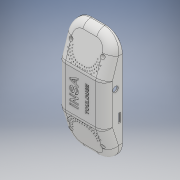
# Autodesk Inventor part: Partie basse
Saved by Autodesk Inventor 2019 (Build 230136000, 136)
## iProperties
Created: 2018-06-04
Part Number: Partie basse
Material: Plastique ABS
Document SubType Name: Modeling
Designer: dimercur
Mass: 82.847 g
Surface Area: 638.157 cm^2
Volume: 78.1576 cm^3
Density: 1.06 g/cm^3
Appearance: Lisse - Blanc
Author: dimercur
Autodesk Inventor part; units mm, degrees
ref_plane "YZ Plane" through (0, 0, 0) normal (1, 0, 0) x (0, 1, 0)
ref_plane "XZ Plane" through (0, 0, 0) normal (0, 1, 0) x (-1, 0, 0)
ref_plane "XY Plane" through (0, 0, 0) normal (0, 0, 1) x (1, 0, 0)
sketch "Esquisse1" plane through (0, 0, 0) normal (0, 1, 0) x (-1, 0, 0)
  line L0 (42.5, 100) -> (-42.5, 100)
  line L1 (-42.5, 100) -> (-42.5, -100)
  line L2 (-42.5, -100) -> (42.5, -100)
  line L3 (42.5, -100) -> (42.5, 100)
  point P0 (0, 0)
  dimension "d0" = 200
  dimension "d1" = 85
  dimension "d2" = 42.5
  dimension "d3" = 100
  constraints: 8 end point, 2 parallel, 1 horizontal, 1 perpendicular
  measures "d0" distance of L2.end L0.start
  measures "d1" distance of L0.start L0.end
  measures "d2" horizontal distance of point (0, 0) L0.start
  measures "d3" vertical distance of point (0, 0) L0.start
extrude "Extrusion1" add sketch "Esquisse1" along normal blind 34
sketch "Esquisse14" plane through (0, 34, 0) normal (0, 1, 0) x (1, 0, 0)
  circle A0 centre (-27.5, -70) radius 3.5
  circle A1 centre (29.5, -70) radius 3.5
  circle A2 centre (29.5, 70) radius 3.5
  circle A3 centre (-27.5, 70) radius 3.5
  line L0 (-42.5, 100) -> (-42.5, -100) projected
  line L1 (42.5, -100) -> (42.5, 100) projected
  line L2 (-42.5, -100) -> (42.5, -100) projected
  line L3 (42.5, 100) -> (-42.5, 100) projected
  point P0 (0, 0)
  dimension "d110" = 7
  dimension "d111" = 7
  dimension "d112" = 7
  dimension "d113" = 7
  dimension "d114" = 15
  dimension "d115" = 15
  dimension "d116" = 13
  dimension "d117" = 13
  dimension "d118" = 30
  dimension "d119" = 30
  dimension "d120" = 30
  dimension "d121" = 30
  constraints: 4 centre point
  measures "d110" diameter of A0
  measures "d111" diameter of A1
  measures "d112" diameter of A2
  measures "d113" diameter of A3
  measures "d114" distance from line of L0 A0.centre
  measures "d115" distance from line of L0 A3.centre
  measures "d116" distance from line of L1 A1.centre
  measures "d117" distance from line of L1 A2.centre
  measures "d118" distance from line of L2 A0.centre
  measures "d119" distance from line of L2 A1.centre
  measures "d120" distance from line of L3 A3.centre
  measures "d121" distance from line of L3 A2.centre
extrude "Extrusion11" cut sketch "Esquisse14" against normal through all contours A0 | A1 | A2 | A3
chamfer "Chanfrein1" distance 20 angle 72 1 edges at (0, 0, 100) measured on face at (0, 0.5, 100)
chamfer "Chanfrein2" distance 20 angle 72 1 edges at (0, 0, -100) measured on face at (0, 0.5, -100)
fillet "Congé3" radius 30 4 edges at (-42.5, 27, 100) (42.5, 27, 100) (-42.5, 27, -100) (42.5, 27, -100)
fillet "Congé4" radius 15 14 edges at (0, 0, 38.4463) (-33.7132, 17.145, 91.2132) (-42.5, 5.1262, 54.2232) (33.7132, 17.145, 91.2132) (42.5, 5.1262, 54.2232) (0, 20, 100) (-42.5, 0, 0) (42.5, 0, 0) (0, 0, -38.4463) (33.7132, 17.145, -91.2132) (42.5, 5.1262, -54.2232) (-33.7132, 17.145, -91.2132) (-42.5, 5.1262, -54.2232) (0, 20, -100)
shell "Coque1" thickness 2.5 removed faces 1 at (10.0863, 34, -22.2425)
sketch "Esquisse3" plane through (0, 34, 0) normal (0, 1, 0) x (1, 0, 0)
  arc A0 (42.5, 70) -> (12.5, 100) centre (12.5, 70) ccw projected
  line L0 (12.5, 100) -> (-12.5, 100) projected
  arc A1 (-12.5, 100) -> (-42.5, 70) centre (-12.5, 70) ccw projected
  line L1 (-42.5, 70) -> (-42.5, -70) projected
  arc A2 (-42.5, -70) -> (-12.5, -100) centre (-12.5, -70) ccw projected
  line L2 (-12.5, -100) -> (12.5, -100) projected
  arc A3 (12.5, -100) -> (42.5, -70) centre (12.5, -70) ccw projected
  line L3 (42.5, -70) -> (42.5, 70) projected
  point P0 (0, 0)
extrude "Extrusion2" add sketch "Esquisse3" along normal blind 2.5
sketch "Esquisse4" plane through (0, 36.5, 0) normal (0, 1, 0) x (1, 0, 0)
  line L0 (35, 54) -> (-35, 54)
  line L1 (-35, 54) -> (-35, -54)
  line L2 (-35, -54) -> (35, -54)
  line L3 (35, -54) -> (35, 54)
  line L4 (27.5, -39.9333) -> (-27.5, -39.9333) projected
  circle A0 centre (-18.5, -39.9333) radius 5
  circle A1 centre (-8.5, -80) radius 5
  circle A2 centre (1.5, -39.9333) radius 5
  circle A3 centre (11.5, -80) radius 5
  circle A4 centre (12.5, 78) radius 5
  circle A5 centre (-12.5, 78) radius 5
  circle A6 centre (0.5, 88) radius 5
  circle A7 centre (0.5, 68) radius 5
  line L5 (42.5, -70) -> (42.5, 70) projected
  line L6 (-42.5, 70) -> (-42.5, -70) projected
  line L7 (12.5, 100) -> (-12.5, 100) projected
  line L8 (-12.5, -100) -> (12.5, -100) projected
  point P0 (0, 0)
  dimension "d19" = 108
  dimension "d20" = 70
  dimension "d21" = 35
  dimension "d22" = 54
  dimension "d23" = 10
  dimension "d24" = 10
  dimension "d25" = 10
  dimension "d26" = 10
  dimension "d27" = 10
  dimension "d28" = 10
  dimension "d29" = 10
  dimension "d30" = 10
  dimension "d31" = 25
  dimension "d32" = 12.5
  dimension "d33" = 20
  dimension "d34" = 42
  dimension "d35" = 42
  dimension "d36" = 30
  dimension "d37" = 22
  dimension "d38" = 24
  dimension "d39" = 20
  dimension "d40" = 20
  dimension "d41" = 20
  dimension "d42" = 20
  dimension "d43" = 34
  dimension "d44" = 12
  constraints: 8 centre point, 8 end point, 2 parallel, 2 point on line, 1 horizontal, 1 perpendicular
  measures "d19" distance of L2.end L0.start
  measures "d20" distance of L0.start L0.end
  measures "d21" horizontal distance of point (0, 0) L0.start
  measures "d22" vertical distance of point (0, 0) L0.start
  measures "d23" diameter of A6
  measures "d24" diameter of A4
  measures "d25" diameter of A7
  measures "d26" diameter of A5
  measures "d27" diameter of A2
  measures "d28" diameter of A3
  measures "d29" diameter of A1
  measures "d30" diameter of A0
  measures "d31" distance of A5.centre A4.centre
  measures "d32" horizontal distance of point (0, 0) A4.centre
  measures "d33" distance of A7.centre A6.centre
  measures "d34" distance from line of L5 A6.centre
  measures "d35" distance from line of L5 A7.centre
  measures "d36" distance from line of L6 A5.centre
  measures "d37" distance from line of L7 A4.centre
  measures "d38" distance from line of L6 A0.centre
  measures "d39" distance of A0.centre A2.centre
  measures "d40" distance of A3.centre A1.centre
  measures "d41" distance from line of L8 A1.centre
  measures "d42" distance from line of L8 A3.centre
  measures "d43" distance from line of L6 A1.centre
  measures "d44" distance from line of L7 A6.centre
extrude "Extrusion3" cut sketch "Esquisse4" against normal blind 3 contours L3 L2 L1 L0 | A2 L4 | L4 A2 | A0 L4 | L4 A0 | A1 | A3 | A4 | A5 | A6 | A7
sketch "Esquisse5" plane through (42.5, 15, 36.0706) normal (1, 0, 0) x (0, 0, -1)
  line L0 (-68.9294, 19) -> (139.0706, 19)
  line L1 (139.0706, 19) -> (139.0706, 27)
  line L2 (139.0706, 27) -> (-68.9294, 27)
  line L3 (-68.9294, 27) -> (-68.9294, 19)
  line L4 (-33.9294, 21.5) -> (-63.9294, 21.5) projected
  line L5 (-63.9294, 21.5) -> (-63.9294, 15.8981) projected
  point P0 (36.0706, -15)
  dimension "d47" = 2.5
  dimension "d48" = 208
  dimension "d49" = 5
  dimension "d50" = 8
  constraints: 8 end point, 2 parallel, 1 horizontal, 1 perpendicular
  measures "d47" distance between parallel lines of L0 L4
  measures "d48" distance of L1.end L2.end
  measures "d49" distance between parallel lines of L5 L3
  measures "d50" distance of L2.end L0.start
extrude "Extrusion4" cut sketch "Esquisse5" against normal through all
sketch "Esquisse6" plane through (42.5, 34, 70) normal (0, 1, 0) x (1, 0, 0)
  line L0 (-85, 0) -> (-85, 140) projected
  arc A0 (-85, 0) -> (-55, -30) centre (-55, 0) ccw projected
  line L1 (-30, -30) -> (-55, -30) projected
  arc A1 (-30, -30) -> (0, 0) centre (-30, 0) ccw projected
  line L2 (0, 140) -> (0, 0) projected
  arc A2 (0, 140) -> (-30, 170) centre (-30, 140) ccw projected
  line L3 (-55, 170) -> (-30, 170) projected
  arc A3 (-55, 170) -> (-85, 140) centre (-55, 140) ccw projected
  line L4 (-83.75, 140) -> (-83.75, 0)
  arc A4 (-83.75, 0) -> (-55, -28.75) centre (-55, 0) ccw
  line L5 (-55, -28.75) -> (-30, -28.75)
  arc A5 (-30, -28.75) -> (-1.25, 0) centre (-30, 0) ccw
  line L6 (-1.25, 0) -> (-1.25, 140)
  arc A6 (-1.25, 140) -> (-30, 168.75) centre (-30, 140) ccw
  line L7 (-30, 168.75) -> (-55, 168.75)
  arc A7 (-55, 168.75) -> (-83.75, 140) centre (-55, 140) ccw
  point P0 (-42.5, 70)
  dimension "d53" = 1.25
  constraints: 8 end point, 8 point on circle, 4 centre point, 7 other
  measures "d53" distance between parallel lines of L4 L0
extrude "Extrusion5" cut sketch "Esquisse6" against normal blind 1
sketch "Esquisse8" plane through (-42.5, 15, -36.0706) normal (-1, 0, 0) x (0, 0, 1)
  line L0 (42.5706, 13.5) -> (61.0706, 13.5)
  line L1 (61.0706, 13.5) -> (61.0706, -1.5)
  line L2 (61.0706, -1.5) -> (42.5706, -1.5)
  line L3 (42.5706, -1.5) -> (42.5706, 13.5)
  line L4 (136.0706, 15.8981) -> (136.0706, 18) projected
  line L5 (106.0706, 18) -> (-33.9294, 18) projected
  point P0 (36.0706, -15)
  dimension "d64" = 18.5
  dimension "d65" = 15
  dimension "d66" = 75
  dimension "d67" = 19.5
  constraints: 8 end point, 2 parallel, 1 horizontal, 1 perpendicular
  measures "d64" distance of L0.start L0.end
  measures "d65" distance of L0.end L1.end
  measures "d66" distance from line of L4 L0.end
  measures "d67" distance between parallel lines of L2 L5
extrude "Extrusion6" cut sketch "Esquisse8" against normal blind 5
sketch "Esquisse9" plane through (-42.5, 15, -36.0706) normal (-1, 0, 0) x (0, 0, 1)
  circle A0 centre (75.9706, 9.9) radius 3.5
  circle A1 centre (86.9706, 9.9) radius 3.5
  line L0 (106.0706, 18) -> (-33.9294, 18) projected
  point P0 (36.0706, -15)
  point P1 (136.0706, 18)
  dimension "d70" = 7
  dimension "d71" = 7
  dimension "d72" = 49.1
  dimension "d73" = 60.1
  dimension "d76" = 8.1
  dimension "d77" = 8.1
  constraints: 2 centre point
  measures "d70" diameter of A0
  measures "d71" diameter of A1
  measures "d72" horizontal distance of point (136.071, 18) A1.centre
  measures "d73" horizontal distance of point (136.071, 18) A0.centre
  measures "d76" distance from line of L0 A0.centre
  measures "d77" vertical distance of point (136.071, 18) A1.centre
extrude "Extrusion7" cut sketch "Esquisse9" against normal blind 5
sketch "Esquisse10" plane through (-42.5, 15, -36.0706) normal (-1, 0, 0) x (0, 0, 1)
  line L0 (-14.4294, 14.5) -> (-2.4294, 14.5)
  line L1 (-2.4294, 14.5) -> (-2.4294, 8)
  line L2 (-2.4294, 8) -> (-14.4294, 8)
  line L3 (-14.4294, 8) -> (-14.4294, 14.5)
  line L4 (6.8706, 14.5) -> (18.8706, 14.5)
  line L5 (18.8706, 14.5) -> (18.8706, 8)
  line L6 (18.8706, 8) -> (6.8706, 8)
  line L7 (6.8706, 8) -> (6.8706, 14.5)
  line L8 (24.4706, 14.5) -> (36.4706, 14.5)
  line L9 (36.4706, 14.5) -> (36.4706, 8)
  line L10 (36.4706, 8) -> (24.4706, 8)
  line L11 (24.4706, 8) -> (24.4706, 14.5)
  line L12 (-63.9294, 18) -> (-63.9294, 15.8981) projected
  line L13 (106.0706, 18) -> (-33.9294, 18) projected
  point P0 (36.0706, -15)
  dimension "d78" = 12
  dimension "d79" = 12
  dimension "d80" = 12
  dimension "d84" = 49.5
  dimension "d85" = 70.8
  dimension "d86" = 88.4
  dimension "d183" = 3.5
  dimension "d184" = 6.5
  dimension "d185" = 6.5
  dimension "d186" = 6.5
  constraints: 24 end point, 4 point on line, 3 horizontal, 3 parallel, 3 perpendicular
  measures "d78" distance of L0.start L0.end
  measures "d79" distance of L4.start L4.end
  measures "d80" distance of L8.start L8.end
  measures "d84" distance between parallel lines of L12 L3
  measures "d85" distance from line of L12.start L7
  measures "d86" distance between parallel lines of L12 L11
  measures "d183" distance between parallel lines of L0 L13
  measures "d184" distance between parallel lines of L2 L0
  measures "d185" distance of L6.end L4.start
  measures "d186" distance of L10.end L8.start
extrude "Extrusion8" cut sketch "Esquisse10" against normal blind 5
sketch "Esquisse11" plane through (42.5, 15, 36.0706) normal (1, 0, 0) x (0, 0, -1)
  line L0 (55.5706, 14.5) -> (71.5706, 14.5)
  line L1 (71.5706, 14.5) -> (71.5706, 11)
  line L2 (71.5706, 11) -> (55.5706, 11)
  line L3 (55.5706, 11) -> (55.5706, 14.5)
  line L4 (106.0706, 18) -> (-33.9294, 18) projected
  point P0 (36.0706, -15)
  point P1 (136.0706, 18)
  dimension "d90" = 3.5
  dimension "d91" = 16
  dimension "d92" = 3.5
  dimension "d93" = 64.5
  constraints: 8 end point, 2 parallel, 1 horizontal, 1 perpendicular
  measures "d90" distance between parallel lines of L2 L0
  measures "d91" distance of L0.start L0.end
  measures "d92" distance between parallel lines of L4 L0
  measures "d93" distance from line of L1 point (136.071, 18)
extrude "Extrusion9" cut sketch "Esquisse11" against normal blind 5
sketch "Esquisse15" plane through (-27.5, 34, 70) normal (0, 1, 0) x (1, 0, 0)
  circle A0 centre (0, 0) radius 6 projected
  circle A1 centre (57, 0) radius 6 projected
  circle A2 centre (57, 140) radius 6 projected
  circle A3 centre (0, 140) radius 6 projected
  point P0 (27.5, 70)
extrude "Extrusion12" cut sketch "Esquisse15" against normal blind 13
sketch "Esquisse16" plane through (-27.5, 21, 70) normal (0, 1, 0) x (1, 0, 0)
  circle A0 centre (0, 0) radius 6 projected
  circle A1 centre (57, 0) radius 6 projected
  circle A2 centre (57, 140) radius 6 projected
  circle A3 centre (0, 140) radius 6 projected
  circle A4 centre (0, 0) radius 1.75
  circle A5 centre (57, 0) radius 1.75
  circle A6 centre (57, 140) radius 1.75
  circle A7 centre (0, 140) radius 1.75
  point P0 (27.5, 70)
  dimension "d126" = 3.5
  dimension "d127" = 3.5
  dimension "d128" = 3.5
  dimension "d129" = 3.5
  constraints: 4 centre point, 4 coincident
  measures "d126" diameter of A4
  measures "d127" diameter of A5
  measures "d128" diameter of A6
  measures "d129" diameter of A7
extrude "Extrusion13" add sketch "Esquisse16" along normal blind 3
sketch "Esquisse17" plane through (0, 0, 0) normal (0, -1, 0) x (1, 0, 0)
  line L0 (-79.1178, 0) -> (59.6619, 0)
  circle A0 centre (-4.5, 46) radius 0.75
  line L1 (12.5, 100) -> (-12.5, 100) projected
  circle A1 centre (-4.5, 64) radius 0.5
  line L2 (-42.5, 70) -> (-42.5, 36.0706) projected
  line L3 (0, 119.1841) -> (0, -113.7497)
  line L4 (-42.5, -36.0706) -> (-42.5, -70) projected
  line L5 (-12.5, -100) -> (12.5, -100) projected
  circle A2 centre (-8.5054, 46.4513) radius 0.75
  circle A3 centre (-12.3099, 47.7826) radius 0.75
  circle A4 centre (-15.7228, 49.927) radius 0.75
  circle A5 centre (-18.573, 52.7772) radius 0.75
  circle A6 centre (-20.7174, 56.1901) radius 0.75
  circle A7 centre (-22.0487, 59.9946) radius 0.75
  circle A8 centre (-22.5, 64) radius 0.75
  circle A9 centre (-6.5, 42) radius 0.75
  circle A10 centre (-10.7139, 42.8012) radius 0.75
  circle A11 centre (-14.6936, 44.4018) radius 0.75
  circle A12 centre (-18.2889, 46.7412) radius 0.75
  circle A13 centre (-21.3643, 49.7313) radius 0.75
  circle A14 centre (-23.8039, 53.2594) radius 0.75
  circle A15 centre (-25.5157, 57.1925) radius 0.75
  circle A16 centre (-26.4351, 61.3822) radius 0.75
  circle A17 centre (-18, 42) radius 0.75
  circle A18 centre (-22.0326, 45.0564) radius 0.75
  circle A19 centre (-25.3914, 48.8409) radius 0.75
  circle A20 centre (-27.9474, 53.2079) radius 0.75
  circle A21 centre (-29.6023, 57.9896) radius 0.75
  circle A22 centre (4.5, 46) radius 0.75
  circle A23 centre (4.5, 64) radius 0.5
  circle A24 centre (8.5054, 46.4513) radius 0.75
  circle A25 centre (12.3099, 47.7826) radius 0.75
  circle A26 centre (15.7228, 49.927) radius 0.75
  circle A27 centre (18.573, 52.7772) radius 0.75
  circle A28 centre (20.7174, 56.1901) radius 0.75
  circle A29 centre (22.0487, 59.9946) radius 0.75
  circle A30 centre (22.5, 64) radius 0.75
  circle A31 centre (6.5, 42) radius 0.75
  circle A32 centre (10.7139, 42.8012) radius 0.75
  circle A33 centre (14.6936, 44.4018) radius 0.75
  circle A34 centre (18.2889, 46.7412) radius 0.75
  circle A35 centre (21.3643, 49.7313) radius 0.75
  circle A36 centre (23.8039, 53.2594) radius 0.75
  circle A37 centre (25.5157, 57.1925) radius 0.75
  circle A38 centre (26.4351, 61.3822) radius 0.75
  circle A39 centre (18, 42) radius 0.75
  circle A40 centre (22.0326, 45.0564) radius 0.75
  circle A41 centre (25.3914, 48.8409) radius 0.75
  circle A42 centre (27.9474, 53.2079) radius 0.75
  circle A43 centre (29.6023, 57.9896) radius 0.75
  circle A44 centre (-4.5, -46) radius 0.75
  circle A45 centre (-4.5, -64) radius 0.5
  circle A46 centre (-8.5054, -46.4513) radius 0.75
  circle A47 centre (-12.3099, -47.7826) radius 0.75
  circle A48 centre (-15.7228, -49.927) radius 0.75
  circle A49 centre (-18.573, -52.7772) radius 0.75
  circle A50 centre (-20.7174, -56.1901) radius 0.75
  circle A51 centre (-22.0487, -59.9946) radius 0.75
  circle A52 centre (-22.5, -64) radius 0.75
  circle A53 centre (-6.5, -42) radius 0.75
  circle A54 centre (-10.7139, -42.8012) radius 0.75
  circle A55 centre (-14.6936, -44.4018) radius 0.75
  circle A56 centre (-18.2889, -46.7412) radius 0.75
  circle A57 centre (-21.3643, -49.7313) radius 0.75
  circle A58 centre (-23.8039, -53.2594) radius 0.75
  circle A59 centre (-25.5157, -57.1925) radius 0.75
  circle A60 centre (-26.4351, -61.3822) radius 0.75
  circle A61 centre (-18, -42) radius 0.75
  circle A62 centre (-22.0326, -45.0564) radius 0.75
  circle A63 centre (-25.3914, -48.8409) radius 0.75
  circle A64 centre (-27.9474, -53.2079) radius 0.75
  circle A65 centre (-29.6023, -57.9896) radius 0.75
  circle A66 centre (15.7228, -49.927) radius 0.75
  circle A67 centre (12.3099, -47.7826) radius 0.75
  circle A68 centre (8.5054, -46.4513) radius 0.75
  circle A69 centre (4.5, -46) radius 0.75
  circle A70 centre (18.2889, -46.7412) radius 0.75
  circle A71 centre (14.6936, -44.4018) radius 0.75
  circle A72 centre (25.3914, -48.8409) radius 0.75
  circle A73 centre (10.7139, -42.8012) radius 0.75
  circle A74 centre (6.5, -42) radius 0.75
  circle A75 centre (22.0326, -45.0564) radius 0.75
  circle A76 centre (18, -42) radius 0.75
  circle A77 centre (21.3643, -49.7313) radius 0.75
  circle A78 centre (18.573, -52.7772) radius 0.75
  circle A79 centre (20.7174, -56.1901) radius 0.75
  circle A80 centre (23.8039, -53.2594) radius 0.75
  circle A81 centre (27.9474, -53.2079) radius 0.75
  circle A82 centre (22.0487, -59.9946) radius 0.75
  circle A83 centre (25.5157, -57.1925) radius 0.75
  circle A84 centre (29.6023, -57.9896) radius 0.75
  circle A85 centre (22.5, -64) radius 0.75
  circle A86 centre (26.4351, -61.3822) radius 0.75
  circle A87 centre (4.5, -64) radius 0.5
  circle A88 centre (0, 45.9912) radius 0.75
  circle A89 centre (0, -45.9912) radius 0.75
  circle A90 centre (-2.5, -42) radius 0.75
  circle A91 centre (2.5, -42) radius 0.75
  circle A92 centre (-2.5, 42) radius 0.75
  circle A93 centre (2.5, 42) radius 0.75
  point P0 (0, 0)
  dimension "d134" = 1.5
  dimension "d135" = 54
  dimension "d136" = 36
  dimension "d138" = 42.5
  dimension "d139" = 100
  dimension "d140" = 38
  dimension "d143" = 90
  dimension "d145" = 38
  dimension "d146" = 1
  dimension "d147" = 1.5
  dimension "d148" = 58
  dimension "d149" = 36
  dimension "d152" = 78
  dimension "d154" = 1.5
  dimension "d155" = 24.5
  dimension "d156" = 58
  dimension "d159" = 45
  dimension "d161" = 1.5
  dimension "d163" = 1.5
  dimension "d164" = 1.5
  dimension "d165" = 1.5
  dimension "d166" = 1.5
  dimension "d167" = 1.5
  dimension "d168" = 4
  dimension "d169" = 4
  dimension "d170" = 4
  dimension "d171" = 4
  constraints: 94 centre point, 66 symmetric about line, 4 end point, 2 point on line, 1 horizontal, 1 vertical, 105 other
  measures "d134" diameter of A0
  measures "d135" distance from line of L1 A0.centre
  measures "d136" distance from line of L1 A1.centre
  measures "d138" distance between parallel lines of L4 L3
  measures "d139" distance between parallel lines of L5 L0
  measures "d140" distance from line of L2 A1.centre
  measures "d145" distance from line of L2 A0.centre
  measures "d146" diameter of A1
  measures "d147" diameter of A9
  measures "d148" distance from line of L1 A9.centre
  measures "d149" distance from line of L2 A9.centre
  measures "d154" diameter of A17
  measures "d155" distance from line of L2 A17.centre
  measures "d156" distance from line of L1 A17.centre
  measures "d161" diameter of A88
  measures "d163" diameter of A89
  measures "d164" diameter of A90
  measures "d165" diameter of A91
  measures "d166" diameter of A92
  measures "d167" diameter of A93
  measures "d168" distance of A92.centre A9.centre
  measures "d169" distance of A31.centre A93.centre
  measures "d170" distance of A90.centre A53.centre
  measures "d171" distance of A74.centre A91.centre
extrude "Extrusion14" cut sketch "Esquisse17" against normal through all contours A0 | A88 L3 | L3 A88 | A89 L3 | L3 A89 | A2 | A3 | A4 | A5 | A6 | A7 | A8 | A9 | A10 | A11 | A12 | A13 | A14 | A15 | A16 | A17 | A18 | A19 | A20 | A21 | A22 | A24 | A25 | A26 | A27 | A28 | A29 | A30 | A31 | A32 | A33 | A34 | A35 | A36 | A37 | A38 | A39 | A40 | A41 | A42 | A43 | A44 | A46 | A47 | A48 | A49 | A50 | A51 | A52 | A53 | A54 | A55 | A56 | A57 | A58 | A59 | A60 | A61 | A62 | A63 | A64 | A65 | A66 | A67 | A68 | A69 | A70 | A71 | A72 | A73 | A74 | A75 | A76 | A77 | A78 | A79 | A80 | A81 | A82 | A83 | A84 | A85 | A86 | A90 | A91 | A92 | A93
sketch "Esquisse7" plane through (0, 0, 0) normal (0, -1, 0) x (1, 0, 0)
  line L0 (-19.727, -25.1957) -> (-19.727, 25.1957) construction
  line L1 (-19.727, 25.1957) -> (-4, 25.1957) construction
  line L2 (-4, 25.1957) -> (-4, -25.1957) construction
  line L3 (-4, -25.1957) -> (-19.727, -25.1957) construction
  line L4 (4, -25.1957) -> (4, 25.1957) construction
  line L5 (4, 25.1957) -> (19.727, 25.1957) construction
  line L6 (19.727, 25.1957) -> (19.727, -25.1957) construction
  line L7 (19.727, -25.1957) -> (4, -25.1957) construction
  line L8 (-4.4755, -23.7666) -> (-19.4755, -23.7666)
  line L9 (-19.4755, -23.7666) -> (-19.4755, -20.7369)
  line L10 (-19.4755, -20.7369) -> (-4.4755, -20.7369)
  line L11 (-4.4755, -20.7369) -> (-4.4755, -23.7666)
  line L12 (-4.4755, -17.8215) -> (-19.4755, -17.8215)
  line L13 (-19.4755, -17.8215) -> (-19.4755, -14.8832)
  line L14 (-19.4755, -14.8832) -> (-9.4145, -8.7209)
  line L15 (-9.4145, -8.7209) -> (-19.4755, -8.7209)
  line L16 (-19.4755, -8.7209) -> (-19.4755, -5.9198)
  line L17 (-19.4755, -5.9198) -> (-4.4755, -5.9198)
  line L18 (-4.4755, -5.9198) -> (-4.4755, -8.9496)
  line L19 (-4.4755, -8.9496) -> (-14.3193, -15.0204)
  line L20 (-14.3193, -15.0204) -> (-4.4755, -15.0204)
  line L21 (-4.4755, -15.0204) -> (-4.4755, -17.8215)
  line L22 (-9.3688, -3.4846) -> (-9.6546, -0.5349)
  spline S0 degree 2 poles (-9.6546, -0.5349) (-8.1683, -0.272) (-6.7735, 1.3629) (-6.7735, 2.7349) knots 0 0 0 1 2 2 2
  spline S1 degree 2 poles (-6.7735, 2.7349) (-6.7735, 4.1983) (-8.0083, 5.6846) (-8.8429, 5.6846) knots 0 0 0 1 2 2 2
  spline S2 degree 2 poles (-8.8429, 5.6846) (-9.3802, 5.6846) (-10.1234, 5.0558) (-10.3978, 4.2783) knots 0 0 0 1 2 2 2
  spline S3 degree 2 poles (-10.3978, 4.2783) (-10.5807, 3.7524) (-11.0494, 1.8546) knots 0 0 0 1 1 1
  spline S4 degree 2 poles (-11.0494, 1.8546) (-11.6554, -0.5806) (-12.5357, -1.5639) knots 0 0 0 1 1 1
  spline S5 degree 2 poles (-12.5357, -1.5639) (-13.7705, -2.9473) (-15.5426, -2.9473) knots 0 0 0 1 1 1
  spline S6 degree 2 poles (-15.5426, -2.9473) (-16.6973, -2.9473) (-18.6866, -1.6439) (-19.727, 0.8027) (-19.727, 2.5291) knots 0 0 0 1 2 3 3 3
  spline S7 degree 2 poles (-19.727, 2.5291) (-19.727, 5.353) (-17.2575, 8.2113) (-15.1882, 8.2799) knots 0 0 0 1 2 2 2
  line L23 (-15.1882, 8.2799) -> (-15.051, 5.2501)
  spline S8 degree 2 poles (-15.051, 5.2501) (-16.2057, 5.0558) (-17.2232, 3.7753) (-17.2232, 2.4948) knots 0 0 0 1 2 2 2
  spline S9 degree 2 poles (-17.2232, 2.4948) (-17.2232, 1.1686) (-16.6859, 0.4254) knots 0 0 0 1 1 1
  spline S10 degree 2 poles (-16.6859, 0.4254) (-16.3315, -0.0547) (-15.7484, -0.0547) knots 0 0 0 1 1 1
  spline S11 degree 2 poles (-15.7484, -0.0547) (-15.2225, -0.0547) (-14.8337, 0.3912) knots 0 0 0 1 1 1
  spline S12 degree 2 poles (-14.8337, 0.3912) (-14.3536, 0.9742) (-13.3132, 5.3988) (-12.2042, 7.5139) (-10.272, 8.7143) (-8.8429, 8.7143) knots 0 0 0 1 2 3 4 4 4
  spline S13 degree 2 poles (-8.8429, 8.7143) (-7.5624, 8.7143) (-5.3101, 7.2852) (-4.2125, 4.6671) (-4.2125, 2.712) knots 0 0 0 1 2 3 3 3
  spline S14 degree 2 poles (-4.2125, 2.712) (-4.2125, -0.1348) (-6.8421, -3.1874) (-9.3688, -3.4846) knots 0 0 0 1 2 2 2
  line L24 (-4.4755, 24.789) -> (-4.4755, 21.4963)
  line L25 (-4.4755, 21.4963) -> (-7.8825, 20.193)
  line L26 (-7.8825, 20.193) -> (-7.8825, 14.2021)
  line L27 (-7.8825, 14.2021) -> (-4.4755, 12.9559)
  line L28 (-4.4755, 12.9559) -> (-4.4755, 9.7433)
  line L29 (-4.4755, 9.7433) -> (-19.4755, 15.5741)
  line L30 (-19.4755, 15.5741) -> (-19.4755, 18.7982)
  line L31 (-19.4755, 18.7982) -> (-4.4755, 24.789)
  line L32 (-10.4206, 19.2212) -> (-15.977, 17.1518)
  line L33 (-15.977, 17.1518) -> (-10.4206, 15.1168)
  line L34 (-10.4206, 15.1168) -> (-10.4206, 19.2212)
  line L35 (14.9112, -21.6848) -> (9.8434, -21.6848)
  line L36 (9.8434, -21.6848) -> (9.8434, -23.4934)
  line L37 (9.8434, -23.4934) -> (8.8112, -23.4934)
  line L38 (8.8112, -23.4934) -> (8.8112, -18.6487)
  line L39 (8.8112, -18.6487) -> (9.8434, -18.6487)
  line L40 (9.8434, -18.6487) -> (9.8434, -20.4527)
  line L41 (9.8434, -20.4527) -> (14.9112, -20.4527)
  line L42 (14.9112, -20.4527) -> (14.9112, -21.6848)
  spline S15 degree 2 poles (11.8984, -18.1001) (10.9685, -18.1001) (10.3362, -17.8211) knots 0 0 0 1 1 1
  spline S16 degree 2 poles (10.3362, -17.8211) (9.8713, -17.6119) (9.1273, -16.8912) (8.9507, -16.4635) knots 0 0 0 1 2 2 2
  spline S17 degree 2 poles (8.9507, -16.4635) (8.7089, -15.8963) (8.7089, -15.1477) knots 0 0 0 1 1 1
  spline S18 degree 2 poles (8.7089, -15.1477) (8.7089, -13.7994) (10.3827, -12.1814) (11.8705, -12.1814) knots 0 0 0 1 2 2 2
  spline S19 degree 2 poles (11.8705, -12.1814) (13.3443, -12.1814) (15.0135, -13.7901) (15.0135, -15.1338) knots 0 0 0 1 2 2 2
  spline S20 degree 2 poles (15.0135, -15.1338) (15.0135, -16.4914) (13.3536, -18.1001) (11.8984, -18.1001) knots 0 0 0 1 2 2 2
  spline S21 degree 2 poles (11.8565, -16.8308) (12.8934, -16.8308) (13.9627, -15.873) (13.9627, -15.1338) knots 0 0 0 1 2 2 2
  spline S22 degree 2 poles (13.9627, -15.1338) (13.9627, -14.3945) (12.9027, -13.4507) (11.8426, -13.4507) knots 0 0 0 1 2 2 2
  spline S23 degree 2 poles (11.8426, -13.4507) (10.7918, -13.4507) (9.7597, -14.3713) (9.7597, -15.1338) knots 0 0 0 1 2 2 2
  spline S24 degree 2 poles (9.7597, -15.1338) (9.7597, -15.8963) (10.8058, -16.8308) (11.8565, -16.8308) knots 0 0 0 1 2 2 2
  line L43 (8.8112, -11.2283) -> (8.8112, -9.9962)
  line L44 (8.8112, -9.9962) -> (12.1169, -9.9962)
  spline S25 degree 2 poles (12.1169, -9.9962) (12.9027, -9.9962) (13.1351, -9.9497) knots 0 0 0 1 1 1
  spline S26 degree 2 poles (13.1351, -9.9497) (13.5071, -9.8707) (13.9627, -9.2755) (13.9627, -8.7595) knots 0 0 0 1 2 2 2
  spline S27 degree 2 poles (13.9627, -8.7595) (13.9627, -8.2387) (13.535, -7.704) (12.912, -7.5971) (12.1866, -7.5971) knots 0 0 0 1 2 3 3 3
  line L45 (12.1866, -7.5971) -> (8.8112, -7.5971)
  line L46 (8.8112, -7.5971) -> (8.8112, -6.365)
  line L47 (8.8112, -6.365) -> (12.0146, -6.365)
  spline S28 degree 2 poles (12.0146, -6.365) (13.1119, -6.365) (14.0185, -6.5649) (14.6415, -7.0996) (15.0135, -8.0016) (15.0135, -8.7223) knots 0 0 0 1 2 3 4 4 4
  spline S29 degree 2 poles (15.0135, -8.7223) (15.0135, -9.5963) (14.609, -10.4983) (13.9674, -11.0237) (13.6094, -11.1074) knots 0 0 0 1 2 3 3 3
  spline S30 degree 2 poles (13.6094, -11.1074) (13.0886, -11.2283) (12.0658, -11.2283) knots 0 0 0 1 1 1
  line L48 (12.0658, -11.2283) -> (8.8112, -11.2283)
  line L49 (14.9112, -5.0306) -> (8.8623, -5.0306)
  line L50 (8.8623, -5.0306) -> (8.8623, -3.7986)
  line L51 (8.8623, -3.7986) -> (13.879, -3.7986)
  line L52 (13.879, -3.7986) -> (13.879, -0.7346)
  line L53 (13.879, -0.7346) -> (14.9112, -0.7346)
  line L54 (14.9112, -0.7346) -> (14.9112, -5.0306)
  spline S31 degree 2 poles (11.8984, -0.1069) (10.9685, -0.1069) (10.3362, 0.172) knots 0 0 0 1 1 1
  spline S32 degree 2 poles (10.3362, 0.172) (9.8713, 0.3813) (9.1273, 1.1019) (8.9507, 1.5296) knots 0 0 0 1 2 2 2
  spline S33 degree 2 poles (8.9507, 1.5296) (8.7089, 2.0969) (8.7089, 2.8454) knots 0 0 0 1 1 1
  spline S34 degree 2 poles (8.7089, 2.8454) (8.7089, 4.1938) (10.3827, 5.8117) (11.8705, 5.8117) knots 0 0 0 1 2 2 2
  spline S35 degree 2 poles (11.8705, 5.8117) (13.3443, 5.8117) (15.0135, 4.203) (15.0135, 2.8594) knots 0 0 0 1 2 2 2
  spline S36 degree 2 poles (15.0135, 2.8594) (15.0135, 1.5018) (13.3536, -0.1069) (11.8984, -0.1069) knots 0 0 0 1 2 2 2
  spline S37 degree 2 poles (11.8565, 1.1623) (12.8934, 1.1623) (13.9627, 2.1201) (13.9627, 2.8594) knots 0 0 0 1 2 2 2
  spline S38 degree 2 poles (13.9627, 2.8594) (13.9627, 3.5986) (12.9027, 4.5425) (11.8426, 4.5425) knots 0 0 0 1 2 2 2
  spline S39 degree 2 poles (11.8426, 4.5425) (10.7918, 4.5425) (9.7597, 3.6219) (9.7597, 2.8594) knots 0 0 0 1 2 2 2
  spline S40 degree 2 poles (9.7597, 2.8594) (9.7597, 2.0969) (10.8058, 1.1623) (11.8565, 1.1623) knots 0 0 0 1 2 2 2
  line L55 (8.8112, 6.7649) -> (8.8112, 7.997)
  line L56 (8.8112, 7.997) -> (12.1169, 7.997)
  spline S41 degree 2 poles (12.1169, 7.997) (12.9027, 7.997) (13.1351, 8.0434) knots 0 0 0 1 1 1
  spline S42 degree 2 poles (13.1351, 8.0434) (13.5071, 8.1225) (13.9627, 8.7176) (13.9627, 9.2337) knots 0 0 0 1 2 2 2
  spline S43 degree 2 poles (13.9627, 9.2337) (13.9627, 9.7544) (13.535, 10.2891) (12.912, 10.396) (12.1866, 10.396) knots 0 0 0 1 2 3 3 3
  line L57 (12.1866, 10.396) -> (8.8112, 10.396)
  line L58 (8.8112, 10.396) -> (8.8112, 11.6281)
  line L59 (8.8112, 11.6281) -> (12.0146, 11.6281)
  spline S44 degree 2 poles (12.0146, 11.6281) (13.1119, 11.6281) (14.0185, 11.4282) (14.6415, 10.8935) (15.0135, 9.9915) (15.0135, 9.2709) knots 0 0 0 1 2 3 4 4 4
  spline S45 degree 2 poles (15.0135, 9.2709) (15.0135, 8.3968) (14.609, 7.4948) (13.9674, 6.9694) (13.6094, 6.8857) knots 0 0 0 1 2 3 3 3
  spline S46 degree 2 poles (13.6094, 6.8857) (13.0886, 6.7649) (12.0658, 6.7649) knots 0 0 0 1 1 1
  line L60 (12.0658, 6.7649) -> (8.8112, 6.7649)
  line L61 (12.9213, 12.6138) -> (12.805, 13.8133)
  spline S47 degree 2 poles (12.805, 13.8133) (13.4094, 13.9203) (13.9767, 14.5851) (13.9767, 15.1431) knots 0 0 0 1 2 2 2
  spline S48 degree 2 poles (13.9767, 15.1431) (13.9767, 15.7382) (13.4745, 16.3426) (13.1351, 16.3426) knots 0 0 0 1 2 2 2
  spline S49 degree 2 poles (13.1351, 16.3426) (12.9166, 16.3426) (12.6144, 16.0869) (12.5028, 15.7707) knots 0 0 0 1 2 2 2
  spline S50 degree 2 poles (12.5028, 15.7707) (12.4284, 15.5569) (12.2378, 14.7851) knots 0 0 0 1 1 1
  spline S51 degree 2 poles (12.2378, 14.7851) (11.9914, 13.7947) (11.6334, 13.3949) knots 0 0 0 1 1 1
  spline S52 degree 2 poles (11.6334, 13.3949) (11.1312, 12.8323) (10.4106, 12.8323) knots 0 0 0 1 1 1
  spline S53 degree 2 poles (10.4106, 12.8323) (9.941, 12.8323) (9.132, 13.3623) (8.7089, 14.3573) (8.7089, 15.0594) knots 0 0 0 1 2 3 3 3
  spline S54 degree 2 poles (8.7089, 15.0594) (8.7089, 16.2078) (9.7132, 17.3701) (10.5547, 17.398) knots 0 0 0 1 2 2 2
  line L62 (10.5547, 17.398) -> (10.6105, 16.1659)
  spline S55 degree 2 poles (10.6105, 16.1659) (10.1409, 16.0869) (9.7271, 15.5662) (9.7271, 15.0454) knots 0 0 0 1 2 2 2
  spline S56 degree 2 poles (9.7271, 15.0454) (9.7271, 14.5061) (9.9456, 14.2039) knots 0 0 0 1 1 1
  spline S57 degree 2 poles (9.9456, 14.2039) (10.0898, 14.0086) (10.3269, 14.0086) knots 0 0 0 1 1 1
  spline S58 degree 2 poles (10.3269, 14.0086) (10.5408, 14.0086) (10.6988, 14.1899) knots 0 0 0 1 1 1
  spline S59 degree 2 poles (10.6988, 14.1899) (10.8941, 14.4271) (11.3172, 16.2264) (11.7682, 17.0865) (12.5539, 17.5747) (13.1351, 17.5747) knots 0 0 0 1 2 3 4 4 4
  spline S60 degree 2 poles (13.1351, 17.5747) (13.6559, 17.5747) (14.5718, 16.9935) (15.0181, 15.9288) (15.0181, 15.1338) knots 0 0 0 1 2 3 3 3
  spline S61 degree 2 poles (15.0181, 15.1338) (15.0181, 13.9761) (13.9488, 12.7347) (12.9213, 12.6138) knots 0 0 0 1 2 2 2
  line L63 (14.9112, 18.6162) -> (8.8112, 18.6162)
  line L64 (8.8112, 18.6162) -> (8.8112, 23.14)
  line L65 (8.8112, 23.14) -> (9.8434, 23.14)
  line L66 (9.8434, 23.14) -> (9.8434, 19.8482)
  line L67 (9.8434, 19.8482) -> (11.1963, 19.8482)
  line L68 (11.1963, 19.8482) -> (11.1963, 22.9122)
  line L69 (11.1963, 22.9122) -> (12.2285, 22.9122)
  line L70 (12.2285, 22.9122) -> (12.2285, 19.8482)
  line L71 (12.2285, 19.8482) -> (13.879, 19.8482)
  line L72 (13.879, 19.8482) -> (13.879, 23.2563)
  line L73 (13.879, 23.2563) -> (14.9112, 23.2563)
  line L74 (14.9112, 23.2563) -> (14.9112, 18.6162)
  point P0 (0, 0)
  dimension "d56" = 50.3915
  dimension "d59" = 25.1957
  dimension "d175" = 15.727
  dimension "d178" = 50.3915
  dimension "d179" = 15.727
  dimension "d180" = 25.1957
  dimension "d181" = 4
  dimension "d182" = 4
  constraints: 4 other
  measures "d56" distance of L0.end L0.start
  measures "d59" vertical distance of point (0, 0) L0.start
  measures "d175" distance of L2.end L0.start
  measures "d178" distance of L7.end L4.end
  measures "d179" distance of L7.start L7.end
  measures "d180" vertical distance of L7.end point (0, 0)
  measures "d181" horizontal distance of point (0, 0) L7.end
  measures "d182" horizontal distance of point (0, 0) L2.end
emboss "Gravure1" sketch "Esquisse7" operation cut depth 1 direction (0, 1, 0)
sketch "Esquisse18" plane through (42.5, 15, 36.0706) normal (1, 0, 0) x (0, 0, -1)
  circle A0 centre (15.5706, 5.5) radius 5
  line L0 (55.5706, 11) -> (55.5706, 14.5) projected
  line L1 (106.0706, 18) -> (-33.9294, 18) projected
  point P0 (36.0706, -15)
  dimension "d187" = 10
  dimension "d188" = 40
  dimension "d189" = 12.5
  constraints: 1 centre point
  measures "d187" diameter of A0
  measures "d188" distance from line of L0 A0.centre
  measures "d189" distance from line of A0.centre L1
extrude "Extrusion15" cut sketch "Esquisse18" against normal blind 10
equation "\"d111\" = d110"
equation "\"d112\" = d110"
equation "\"d113\" = d110"
equation "\"d115\" = d114"
equation "\"d117\" = d116"
equation "\"d118\" = d119"
equation "\"d120\" = d118"
equation "\"d121\" = d119"
equation "\"d21\" = 0.5 * d20"
equation "\"d22\" = 0.5 * d19"
equation "\"d32\" = 0.5 * d31"
equation "\"d71\" = d70"
equation "\"d77\" = d76"
equation "\"d79\" = d78"
equation "\"d80\" = d78"
equation "\"d127\" = d126"
equation "\"d128\" = d126"
equation "\"d129\" = d126"
equation "\"d2\" = 0.5 * d1"
equation "\"d3\" = 0.5 * d0"
equation "\"d59\" = 0.5 * d56"
